Autodesk Inventor part; units mm, degrees
(part 2 of 2)
  spline S96 degree 3 poles (14.7882, -6.4465) (14.7882, -5.3187) (15.0875, -4.3953) (15.6861, -3.6762) knots 0 0 0 0 1 1 1 1
  line L430 (14.7882, -6.4465) -> (14.7882, -5.3187) construction
  line L431 (14.7882, -5.3187) -> (15.0875, -4.3953) construction
  line L432 (15.0875, -4.3953) -> (15.6861, -3.6762) construction
  spline S97 degree 3 poles (15.6861, -3.6762) (16.2847, -2.9572) (17.1023, -2.5977) (18.1388, -2.5977) knots 0 0 0 0 1 1 1 1
  line L433 (15.6861, -3.6762) -> (16.2847, -2.9572) construction
  line L434 (16.2847, -2.9572) -> (17.1023, -2.5977) construction
  line L435 (17.1023, -2.5977) -> (18.1388, -2.5977) construction
  spline S98 degree 3 poles (18.1388, -2.5977) (19.9346, -2.5977) (20.9456, -3.5631) (21.1719, -5.4939) knots 0 0 0 0 1 1 1 1
  line L436 (18.1388, -2.5977) -> (19.9346, -2.5977) construction
  line L437 (19.9346, -2.5977) -> (20.9456, -3.5631) construction
  line L438 (20.9456, -3.5631) -> (21.1719, -5.4939) construction
  line L439 (19.4747, -7.4594) -> (21.1719, -7.5634)
  line L440 (27.9553, -2.7127) -> (27.9553, -10.1858)
  line L441 (27.9553, -10.1858) -> (26.2362, -10.1858)
  line L442 (26.2362, -10.1858) -> (26.2362, -7.1035)
  line L443 (26.2362, -7.1035) -> (23.8984, -7.1035)
  line L444 (23.8984, -7.1035) -> (23.8984, -10.1858)
  line L445 (23.8984, -10.1858) -> (22.1793, -10.1858)
  line L446 (22.1793, -10.1858) -> (22.1793, -2.7127)
  line L447 (22.1793, -2.7127) -> (23.8984, -2.7127)
  line L448 (23.8984, -2.7127) -> (23.8984, -5.6253)
  line L449 (23.8984, -5.6253) -> (26.2362, -5.6253)
  line L450 (26.2362, -5.6253) -> (26.2362, -2.7127)
  line L451 (26.2362, -2.7127) -> (27.9553, -2.7127)
  line L452 (-87.9456, 18.7555) -> (-34.3787, 18.7555) construction
  line L453 (-34.3787, 18.7555) -> (-34.3787, -19.0126) construction
  line L454 (-34.3787, -19.0126) -> (-87.9456, -19.0126) construction
  line L455 (-87.9456, -19.0126) -> (-87.9456, 18.7555) construction
  line L456 (-69.5997, 11.0371) -> (-69.5997, 16.9868)
  line L457 (-69.5997, 16.9868) -> (-68.3878, 16.9868)
  line L458 (-68.3878, 16.9868) -> (-68.3878, 12.0523)
  line L459 (-68.3878, 12.0523) -> (-65.3741, 12.0523)
  line L460 (-65.3741, 12.0523) -> (-65.3741, 11.0371)
  line L461 (-65.3741, 11.0371) -> (-69.5997, 11.0371)
  spline S99 degree 2 poles (-64.7567, 14.0005) (-64.7567, 14.9151) (-64.4823, 15.5371) knots 0 0 0 1 1 1
  spline S100 degree 2 poles (-64.4823, 15.5371) (-64.2765, 15.9944) (-63.5677, 16.7261) (-63.1469, 16.8999) knots 0 0 0 1 2 2 2
  spline S101 degree 2 poles (-63.1469, 16.8999) (-62.589, 17.1377) (-61.8527, 17.1377) knots 0 0 0 1 1 1
  spline S102 degree 2 poles (-61.8527, 17.1377) (-60.5265, 17.1377) (-58.935, 15.4914) (-58.935, 14.0279) knots 0 0 0 1 2 2 2
  spline S103 degree 2 poles (-58.935, 14.0279) (-58.935, 12.5783) (-60.5174, 10.9365) (-61.839, 10.9365) knots 0 0 0 1 2 2 2
  spline S104 degree 2 poles (-61.839, 10.9365) (-63.1744, 10.9365) (-64.7567, 12.5691) (-64.7567, 14.0005) knots 0 0 0 1 2 2 2
  spline S105 degree 2 poles (-63.5082, 14.0417) (-63.5082, 13.0218) (-62.5661, 11.97) (-61.839, 11.97) knots 0 0 0 1 2 2 2
  spline S106 degree 2 poles (-61.839, 11.97) (-61.1119, 11.97) (-60.1835, 13.0127) (-60.1835, 14.0554) knots 0 0 0 1 2 2 2
  spline S107 degree 2 poles (-60.1835, 14.0554) (-60.1835, 15.0889) (-61.089, 16.1042) (-61.839, 16.1042) knots 0 0 0 1 2 2 2
  spline S108 degree 2 poles (-61.839, 16.1042) (-62.589, 16.1042) (-63.5082, 15.0752) (-63.5082, 14.0417) knots 0 0 0 1 2 2 2
  line L462 (-55.1988, 13.2368) -> (-55.1988, 14.252)
  line L463 (-55.1988, 14.252) -> (-52.5875, 14.252)
  line L464 (-52.5875, 14.252) -> (-52.5875, 11.8648)
  spline S109 degree 2 poles (-52.5875, 11.8648) (-52.967, 11.4944) (-54.4122, 10.9365) (-55.153, 10.9365) knots 0 0 0 1 2 2 2
  spline S110 degree 2 poles (-55.153, 10.9365) (-56.0951, 10.9365) (-57.4945, 11.7276) (-58.1988, 13.1956) (-58.1988, 14.0554) knots 0 0 0 1 2 3 3 3
  spline S111 degree 2 poles (-58.1988, 14.0554) (-58.1988, 14.9929) (-57.4122, 16.4517) (-56.6576, 16.8404) knots 0 0 0 1 2 2 2
  spline S112 degree 2 poles (-56.6576, 16.8404) (-56.0768, 17.1377) (-55.217, 17.1377) knots 0 0 0 1 1 1
  spline S113 degree 2 poles (-55.217, 17.1377) (-54.1012, 17.1377) (-52.8436, 16.2002) (-52.6652, 15.3725) knots 0 0 0 1 2 2 2
  line L465 (-52.6652, 15.3725) -> (-53.868, 15.1484)
  spline S114 degree 2 poles (-53.868, 15.1484) (-53.996, 15.592) (-54.6957, 16.1042) (-55.217, 16.1042) knots 0 0 0 1 2 2 2
  spline S115 degree 2 poles (-55.217, 16.1042) (-56.0128, 16.1042) (-56.9503, 15.0981) (-56.9503, 14.1057) knots 0 0 0 1 2 2 2
  spline S116 degree 2 poles (-56.9503, 14.1057) (-56.9503, 13.0401) (-55.9991, 11.97) (-55.2308, 11.97) knots 0 0 0 1 2 2 2
  spline S117 degree 2 poles (-55.2308, 11.97) (-54.8512, 11.97) (-54.0875, 12.2673) (-53.8131, 12.4776) knots 0 0 0 1 2 2 2
  line L466 (-53.8131, 12.4776) -> (-53.8131, 13.2368)
  line L467 (-53.8131, 13.2368) -> (-55.1988, 13.2368)
  line L468 (-80.8131, 1.5949) -> (-80.8131, 7.5949)
  line L469 (-80.8131, 7.5949) -> (-78.8695, 7.5949)
  spline S118 degree 2 poles (-78.8695, 7.5949) (-77.7628, 7.5949) (-77.4289, 7.5034) knots 0 0 0 1 1 1
  spline S119 degree 2 poles (-77.4289, 7.5034) (-76.9122, 7.3708) (-76.217, 6.4653) (-76.217, 5.7473) knots 0 0 0 1 2 2 2
  spline S120 degree 2 poles (-76.217, 5.7473) (-76.217, 5.1985) (-76.6195, 4.444) (-77.2369, 4.0141) (-77.557, 3.9455) knots 0 0 0 1 2 3 3 3
  spline S121 degree 2 poles (-77.557, 3.9455) (-77.9869, 3.8586) (-78.81, 3.8586) knots 0 0 0 1 1 1
  line L470 (-78.81, 3.8586) -> (-79.6012, 3.8586)
  line L471 (-79.6012, 3.8586) -> (-79.6012, 1.5949)
  line L472 (-79.6012, 1.5949) -> (-80.8131, 1.5949)
  line L473 (-79.6012, 6.5796) -> (-79.6012, 4.8738)
  line L474 (-79.6012, 4.8738) -> (-78.9381, 4.8738)
  spline S122 degree 2 poles (-78.9381, 4.8738) (-78.2201, 4.8738) (-77.7399, 5.0613) (-77.4655, 5.4638) (-77.4655, 5.729) knots 0 0 0 1 2 3 3 3
  spline S123 degree 2 poles (-77.4655, 5.729) (-77.4655, 6.0583) (-77.8497, 6.4836) (-78.1469, 6.5385) knots 0 0 0 1 2 2 2
  spline S124 degree 2 poles (-78.1469, 6.5385) (-78.3619, 6.5796) (-79.0158, 6.5796) knots 0 0 0 1 1 1
  line L475 (-79.0158, 6.5796) -> (-79.6012, 6.5796)
  line L476 (-75.2201, 1.5949) -> (-75.2201, 7.5949)
  line L477 (-75.2201, 7.5949) -> (-70.7704, 7.5949)
  line L478 (-70.7704, 7.5949) -> (-70.7704, 6.5796)
  line L479 (-70.7704, 6.5796) -> (-74.0082, 6.5796)
  line L480 (-74.0082, 6.5796) -> (-74.0082, 5.2488)
  line L481 (-74.0082, 5.2488) -> (-70.9945, 5.2488)
  line L482 (-70.9945, 5.2488) -> (-70.9945, 4.2336)
  line L483 (-70.9945, 4.2336) -> (-74.0082, 4.2336)
  line L484 (-74.0082, 4.2336) -> (-74.0082, 2.6101)
  line L485 (-74.0082, 2.6101) -> (-70.6561, 2.6101)
  line L486 (-70.6561, 2.6101) -> (-70.6561, 1.5949)
  line L487 (-70.6561, 1.5949) -> (-75.2201, 1.5949)
  line L488 (-69.6271, 1.5949) -> (-69.6271, 7.5949)
  line L489 (-69.6271, 7.5949) -> (-67.0753, 7.5949)
  spline S125 degree 2 poles (-67.0753, 7.5949) (-66.1103, 7.5949) (-65.2414, 7.2702) (-64.7155, 6.447) (-64.7155, 5.912) knots 0 0 0 1 2 3 3 3
  spline S126 degree 2 poles (-64.7155, 5.912) (-64.7155, 5.2397) (-65.5067, 4.3571) (-66.2978, 4.2427) knots 0 0 0 1 2 2 2
  spline S127 degree 2 poles (-66.2978, 4.2427) (-65.9045, 4.0141) (-65.3924, 3.4653) (-64.9579, 2.7656) knots 0 0 0 1 2 2 2
  line L490 (-64.9579, 2.7656) -> (-64.2262, 1.5949)
  line L491 (-64.2262, 1.5949) -> (-65.6759, 1.5949)
  line L492 (-65.6759, 1.5949) -> (-66.5494, 2.9028)
  spline S128 degree 2 poles (-66.5494, 2.9028) (-67.0204, 3.6025) (-67.3634, 3.9684) (-67.7475, 4.101) (-68.1683, 4.101) knots 0 0 0 1 2 3 3 3
  line L493 (-68.1683, 4.101) -> (-68.4152, 4.101)
  line L494 (-68.4152, 4.101) -> (-68.4152, 1.5949)
  line L495 (-68.4152, 1.5949) -> (-69.6271, 1.5949)
  line L496 (-68.4152, 5.0568) -> (-67.5189, 5.0568)
  spline S129 degree 2 poles (-67.5189, 5.0568) (-66.6454, 5.0568) (-66.2109, 5.2031) (-65.964, 5.5644) (-65.964, 5.8342) knots 0 0 0 1 2 3 3 3
  spline S130 degree 2 poles (-65.964, 5.8342) (-65.964, 6.136) (-66.2887, 6.511) (-66.5814, 6.5613) knots 0 0 0 1 2 2 2
  spline S131 degree 2 poles (-66.5814, 6.5613) (-66.7323, 6.5796) (-67.4686, 6.5796) knots 0 0 0 1 1 1
  line L497 (-67.4686, 6.5796) -> (-68.4152, 6.5796)
  line L498 (-68.4152, 6.5796) -> (-68.4152, 5.0568)
  line L499 (-63.6134, 1.5949) -> (-63.6134, 7.5949)
  line L500 (-63.6134, 7.5949) -> (-62.4015, 7.5949)
  line L501 (-62.4015, 7.5949) -> (-62.4015, 1.5949)
  line L502 (-62.4015, 1.5949) -> (-63.6134, 1.5949)
  spline S132 degree 2 poles (-61.4914, 4.5583) (-61.4914, 5.4729) (-61.217, 6.0949) knots 0 0 0 1 1 1
  spline S133 degree 2 poles (-61.217, 6.0949) (-61.0113, 6.5522) (-60.3024, 7.2839) (-59.8817, 7.4577) knots 0 0 0 1 2 2 2
  spline S134 degree 2 poles (-59.8817, 7.4577) (-59.3238, 7.6955) (-58.5875, 7.6955) knots 0 0 0 1 1 1
  spline S135 degree 2 poles (-58.5875, 7.6955) (-57.2613, 7.6955) (-55.6698, 6.0491) (-55.6698, 4.5857) knots 0 0 0 1 2 2 2
  spline S136 degree 2 poles (-55.6698, 4.5857) (-55.6698, 3.136) (-57.2521, 1.4943) (-58.5738, 1.4943) knots 0 0 0 1 2 2 2
  spline S137 degree 2 poles (-58.5738, 1.4943) (-59.9091, 1.4943) (-61.4914, 3.1269) (-61.4914, 4.5583) knots 0 0 0 1 2 2 2
  spline S138 degree 2 poles (-60.243, 4.5995) (-60.243, 3.5796) (-59.3009, 2.5278) (-58.5738, 2.5278) knots 0 0 0 1 2 2 2
  spline S139 degree 2 poles (-58.5738, 2.5278) (-57.8466, 2.5278) (-56.9183, 3.5705) (-56.9183, 4.6132) knots 0 0 0 1 2 2 2
  spline S140 degree 2 poles (-56.9183, 4.6132) (-56.9183, 5.6467) (-57.8238, 6.662) (-58.5738, 6.662) knots 0 0 0 1 2 2 2
  spline S141 degree 2 poles (-58.5738, 6.662) (-59.3238, 6.662) (-60.243, 5.633) (-60.243, 4.5995) knots 0 0 0 1 2 2 2
  line L503 (-54.7323, 7.5949) -> (-52.5143, 7.5949)
  spline S142 degree 2 poles (-52.5143, 7.5949) (-51.7643, 7.5949) (-51.371, 7.4805) knots 0 0 0 1 1 1
  spline S143 degree 2 poles (-51.371, 7.4805) (-50.8451, 7.3251) (-50.0905, 6.5293) (-49.6972, 5.3815) (-49.6972, 4.5354) knots 0 0 0 1 2 3 3 3
  spline S144 degree 2 poles (-49.6972, 4.5354) (-49.6972, 3.7946) (-49.8802, 3.2595) knots 0 0 0 1 1 1
  spline S145 degree 2 poles (-49.8802, 3.2595) (-50.1088, 2.6055) (-50.525, 2.1985) knots 0 0 0 1 1 1
  spline S146 degree 2 poles (-50.525, 2.1985) (-50.8405, 1.8921) (-51.3756, 1.7229) knots 0 0 0 1 1 1
  spline S147 degree 2 poles (-51.3756, 1.7229) (-51.778, 1.5949) (-52.4503, 1.5949) knots 0 0 0 1 1 1
  line L504 (-52.4503, 1.5949) -> (-54.7323, 1.5949)
  line L505 (-54.7323, 1.5949) -> (-54.7323, 7.5949)
  line L506 (-53.5204, 6.5796) -> (-53.5204, 2.6101)
  line L507 (-53.5204, 2.6101) -> (-52.6149, 2.6101)
  spline S148 degree 2 poles (-52.6149, 2.6101) (-52.1027, 2.6101) (-51.8786, 2.6696) knots 0 0 0 1 1 1
  spline S149 degree 2 poles (-51.8786, 2.6696) (-51.5814, 2.7427) (-51.1927, 3.0903) (-50.9457, 3.8998) (-50.9457, 4.5949) knots 0 0 0 1 2 3 3 3
  spline S150 degree 2 poles (-50.9457, 4.5949) (-50.9457, 5.29) (-51.1927, 6.0309) (-51.6363, 6.447) (-51.9747, 6.5202) knots 0 0 0 1 2 3 3 3
  spline S151 degree 2 poles (-51.9747, 6.5202) (-52.2308, 6.5796) (-52.9762, 6.5796) knots 0 0 0 1 1 1
  line L508 (-52.9762, 6.5796) -> (-53.5204, 6.5796)
  line L509 (-48.7094, 1.5949) -> (-48.7094, 7.5949)
  line L510 (-48.7094, 7.5949) -> (-47.4975, 7.5949)
  line L511 (-47.4975, 7.5949) -> (-47.4975, 1.5949)
  line L512 (-47.4975, 1.5949) -> (-48.7094, 1.5949)
  line L513 (-42.5036, 3.8037) -> (-41.3283, 3.4333)
  spline S152 degree 2 poles (-41.3283, 3.4333) (-41.5981, 2.4501) (-42.8558, 1.4943) (-43.8207, 1.4943) knots 0 0 0 1 2 2 2
  spline S153 degree 2 poles (-43.8207, 1.4943) (-45.0143, 1.4943) (-46.5555, 3.1269) (-46.5555, 4.54) knots 0 0 0 1 2 2 2
  spline S154 degree 2 poles (-46.5555, 4.54) (-46.5555, 6.04) (-45.0097, 7.6955) (-43.7475, 7.6955) knots 0 0 0 1 2 2 2
  spline S155 degree 2 poles (-43.7475, 7.6955) (-42.65, 7.6955) (-41.9594, 7.0461) knots 0 0 0 1 1 1
  spline S156 degree 2 poles (-41.9594, 7.0461) (-41.5524, 6.662) (-41.3466, 5.944) knots 0 0 0 1 1 1
  line L514 (-41.3466, 5.944) -> (-42.5448, 5.6559)
  spline S157 degree 2 poles (-42.5448, 5.6559) (-42.65, 6.1223) (-43.3268, 6.662) (-43.807, 6.662) knots 0 0 0 1 2 2 2
  spline S158 degree 2 poles (-43.807, 6.662) (-44.4747, 6.662) (-45.307, 5.7062) (-45.307, 4.6315) knots 0 0 0 1 2 2 2
  spline S159 degree 2 poles (-45.307, 4.6315) (-45.307, 3.4927) (-44.4884, 2.5278) (-43.8344, 2.5278) knots 0 0 0 1 2 2 2
  spline S160 degree 2 poles (-43.8344, 2.5278) (-43.3497, 2.5278) (-42.6545, 3.1452) (-42.5036, 3.8037) knots 0 0 0 1 2 2 2
  line L515 (-75.6385, -7.8473) -> (-76.9556, -7.8473)
  line L516 (-76.9556, -7.8473) -> (-77.477, -6.4845)
  line L517 (-77.477, -6.4845) -> (-79.8733, -6.4845)
  line L518 (-79.8733, -6.4845) -> (-80.3718, -7.8473)
  line L519 (-80.3718, -7.8473) -> (-81.6568, -7.8473)
  line L520 (-81.6568, -7.8473) -> (-79.3245, -1.8473)
  line L521 (-79.3245, -1.8473) -> (-78.0349, -1.8473)
  line L522 (-78.0349, -1.8473) -> (-75.6385, -7.8473)
  line L523 (-77.8657, -5.4693) -> (-78.6934, -3.2467)
  line L524 (-78.6934, -3.2467) -> (-79.5074, -5.4693)
  line L525 (-79.5074, -5.4693) -> (-77.8657, -5.4693)
  line L526 (-74.98, -7.8473) -> (-74.98, -1.8473)
  line L527 (-74.98, -1.8473) -> (-73.8047, -1.8473)
  line L528 (-73.8047, -1.8473) -> (-71.3398, -5.8717)
  line L529 (-71.3398, -5.8717) -> (-71.3398, -1.8473)
  line L530 (-71.3398, -1.8473) -> (-70.2193, -1.8473)
  line L531 (-70.2193, -1.8473) -> (-70.2193, -7.8473)
  line L532 (-70.2193, -7.8473) -> (-71.4312, -7.8473)
  line L533 (-71.4312, -7.8473) -> (-73.8596, -3.9098)
  line L534 (-73.8596, -3.9098) -> (-73.8596, -7.8473)
  line L535 (-73.8596, -7.8473) -> (-74.98, -7.8473)
  line L536 (-67.5852, -7.8473) -> (-67.5852, -2.8626)
  line L537 (-67.5852, -2.8626) -> (-69.3641, -2.8626)
  line L538 (-69.3641, -2.8626) -> (-69.3641, -1.8473)
  line L539 (-69.3641, -1.8473) -> (-64.5989, -1.8473)
  line L540 (-64.5989, -1.8473) -> (-64.5989, -2.8626)
  line L541 (-64.5989, -2.8626) -> (-66.3733, -2.8626)
  line L542 (-66.3733, -2.8626) -> (-66.3733, -7.8473)
  line L543 (-66.3733, -7.8473) -> (-67.5852, -7.8473)
  line L544 (-63.8123, -7.8473) -> (-63.8123, -1.8473)
  line L545 (-63.8123, -1.8473) -> (-59.3626, -1.8473)
  line L546 (-59.3626, -1.8473) -> (-59.3626, -2.8626)
  line L547 (-59.3626, -2.8626) -> (-62.6004, -2.8626)
  line L548 (-62.6004, -2.8626) -> (-62.6004, -4.1934)
  line L549 (-62.6004, -4.1934) -> (-59.5867, -4.1934)
  line L550 (-59.5867, -4.1934) -> (-59.5867, -5.2086)
  line L551 (-59.5867, -5.2086) -> (-62.6004, -5.2086)
  line L552 (-62.6004, -5.2086) -> (-62.6004, -6.8321)
  line L553 (-62.6004, -6.8321) -> (-59.2483, -6.8321)
  line L554 (-59.2483, -6.8321) -> (-59.2483, -7.8473)
  line L555 (-59.2483, -7.8473) -> (-63.8123, -7.8473)
  line L556 (-58.2102, -7.8473) -> (-58.2102, -1.8473)
  line L557 (-58.2102, -1.8473) -> (-57.0349, -1.8473)
  line L558 (-57.0349, -1.8473) -> (-54.5699, -5.8717)
  line L559 (-54.5699, -5.8717) -> (-54.5699, -1.8473)
  line L560 (-54.5699, -1.8473) -> (-53.4495, -1.8473)
  line L561 (-53.4495, -1.8473) -> (-53.4495, -7.8473)
  line L562 (-53.4495, -7.8473) -> (-54.6614, -7.8473)
  line L563 (-54.6614, -7.8473) -> (-57.0898, -3.9098)
  line L564 (-57.0898, -3.9098) -> (-57.0898, -7.8473)
  line L565 (-57.0898, -7.8473) -> (-58.2102, -7.8473)
  line L566 (-52.1553, -7.8473) -> (-52.1553, -1.8473)
  line L567 (-52.1553, -1.8473) -> (-50.98, -1.8473)
  line L568 (-50.98, -1.8473) -> (-48.5151, -5.8717)
  line L569 (-48.5151, -5.8717) -> (-48.5151, -1.8473)
  line L570 (-48.5151, -1.8473) -> (-47.3946, -1.8473)
  line L571 (-47.3946, -1.8473) -> (-47.3946, -7.8473)
  line L572 (-47.3946, -7.8473) -> (-48.6065, -7.8473)
  line L573 (-48.6065, -7.8473) -> (-51.0349, -3.9098)
  line L574 (-51.0349, -3.9098) -> (-51.0349, -7.8473)
  line L575 (-51.0349, -7.8473) -> (-52.1553, -7.8473)
  line L576 (-40.7041, -7.8473) -> (-42.0212, -7.8473)
  line L577 (-42.0212, -7.8473) -> (-42.5425, -6.4845)
  line L578 (-42.5425, -6.4845) -> (-44.9388, -6.4845)
  line L579 (-44.9388, -6.4845) -> (-45.4373, -7.8473)
  line L580 (-45.4373, -7.8473) -> (-46.7224, -7.8473)
  line L581 (-46.7224, -7.8473) -> (-44.3901, -1.8473)
  line L582 (-44.3901, -1.8473) -> (-43.1004, -1.8473)
  line L583 (-43.1004, -1.8473) -> (-40.7041, -7.8473)
  line L584 (-42.9312, -5.4693) -> (-43.759, -3.2467)
  line L585 (-43.759, -3.2467) -> (-44.573, -5.4693)
  line L586 (-44.573, -5.4693) -> (-42.9312, -5.4693)
  spline S161 degree 2 poles (-80.2872, -11.2667) (-79.4137, -11.2667) (-78.9244, -11.8886) knots 0 0 0 1 1 1
  spline S162 degree 2 poles (-78.9244, -11.8886) (-78.339, -12.6249) (-78.339, -14.3307) knots 0 0 0 1 1 1
  spline S163 degree 2 poles (-78.339, -14.3307) (-78.339, -16.0319) (-78.9289, -16.7774) knots 0 0 0 1 1 1
  spline S164 degree 2 poles (-78.9289, -16.7774) (-79.4137, -17.3902) (-80.2872, -17.3902) knots 0 0 0 1 1 1
  spline S165 degree 2 poles (-80.2872, -17.3902) (-81.1652, -17.3902) (-82.2353, -16.0456) (-82.2353, -14.317) knots 0 0 0 1 2 2 2
  spline S166 degree 2 poles (-82.2353, -14.317) (-82.2353, -12.6249) (-81.6454, -11.8795) knots 0 0 0 1 1 1
  spline S167 degree 2 poles (-81.6454, -11.8795) (-81.1606, -11.2667) (-80.2872, -11.2667) knots 0 0 0 1 1 1
  spline S168 degree 2 poles (-80.2872, -12.2225) (-80.4975, -12.2225) (-80.8222, -12.4877) (-80.9137, -12.8307) knots 0 0 0 1 2 2 2
  spline S169 degree 2 poles (-80.9137, -12.8307) (-81.0326, -13.2743) (-81.0326, -14.3307) knots 0 0 0 1 1 1
  spline S170 degree 2 poles (-81.0326, -14.3307) (-81.0326, -15.3825) (-80.8177, -16.1737) (-80.4975, -16.4344) (-80.2872, -16.4344) knots 0 0 0 1 2 3 3 3
  spline S171 degree 2 poles (-80.2872, -16.4344) (-80.0768, -16.4344) (-79.7521, -16.1691) (-79.6606, -15.8261) knots 0 0 0 1 2 2 2
  spline S172 degree 2 poles (-79.6606, -15.8261) (-79.5417, -15.3825) (-79.5417, -14.3307) knots 0 0 0 1 1 1
  spline S173 degree 2 poles (-79.5417, -14.3307) (-79.5417, -13.2743) (-79.7567, -12.4877) (-80.0768, -12.2225) (-80.2872, -12.2225) knots 0 0 0 1 2 3 3 3
  line L587 (-77.3283, -17.2896) -> (-77.3283, -16.1371)
  line L588 (-77.3283, -16.1371) -> (-76.1759, -16.1371)
  line L589 (-76.1759, -16.1371) -> (-76.1759, -17.2896)
  line L590 (-76.1759, -17.2896) -> (-77.3283, -17.2896)
  spline S174 degree 2 poles (-74.2597, -14.0517) (-74.7033, -13.8642) (-75.1103, -13.2057) (-75.1103, -12.8124) knots 0 0 0 1 2 2 2
  spline S175 degree 2 poles (-75.1103, -12.8124) (-75.1103, -12.1402) (-74.1728, -11.2667) (-73.3085, -11.2667) knots 0 0 0 1 2 2 2
  spline S176 degree 2 poles (-73.3085, -11.2667) (-72.4533, -11.2667) (-71.5067, -12.1402) (-71.5067, -12.8124) knots 0 0 0 1 2 2 2
  spline S177 degree 2 poles (-71.5067, -12.8124) (-71.5067, -13.2286) (-71.9411, -13.878) (-72.3344, -14.0517) knots 0 0 0 1 2 2 2
  spline S178 degree 2 poles (-72.3344, -14.0517) (-71.8359, -14.253) (-71.3146, -15.0213) (-71.3146, -15.5243) knots 0 0 0 1 2 2 2
  spline S179 degree 2 poles (-71.3146, -15.5243) (-71.3146, -16.3566) (-72.3756, -17.3947) (-73.2536, -17.3947) knots 0 0 0 1 2 2 2
  spline S180 degree 2 poles (-73.2536, -17.3947) (-74.0722, -17.3947) (-74.6164, -16.9649) knots 0 0 0 1 1 1
  spline S181 degree 2 poles (-74.6164, -16.9649) (-75.2613, -16.4572) (-75.2613, -15.5746) knots 0 0 0 1 1 1
  spline S182 degree 2 poles (-75.2613, -15.5746) (-75.2613, -15.0853) (-74.7765, -14.2713) (-74.2597, -14.0517) knots 0 0 0 1 2 2 2
  spline S183 degree 2 poles (-74.1271, -15.4649) (-74.1271, -15.9405) (-73.6424, -16.471) (-73.2765, -16.471) knots 0 0 0 1 2 2 2
  spline S184 degree 2 poles (-73.2765, -16.471) (-72.9198, -16.471) (-72.4533, -15.9588) (-72.4533, -15.474) knots 0 0 0 1 2 2 2
  spline S185 degree 2 poles (-72.4533, -15.474) (-72.4533, -15.0533) (-72.9289, -14.5411) (-73.2902, -14.5411) knots 0 0 0 1 2 2 2
  spline S186 degree 2 poles (-73.2902, -14.5411) (-73.7155, -14.5411) (-74.1271, -15.1219) (-74.1271, -15.4649) knots 0 0 0 1 2 2 2
  spline S187 degree 2 poles (-74.0219, -12.8947) (-74.0219, -13.2377) (-73.6332, -13.6219) (-73.3085, -13.6219) knots 0 0 0 1 2 2 2
  spline S188 degree 2 poles (-73.3085, -13.6219) (-72.9792, -13.6219) (-72.5859, -13.2331) (-72.5859, -12.8902) knots 0 0 0 1 2 2 2
  spline S189 degree 2 poles (-72.5859, -12.8902) (-72.5859, -12.57) (-72.9747, -12.1813) (-73.2948, -12.1813) knots 0 0 0 1 2 2 2
  spline S190 degree 2 poles (-73.2948, -12.1813) (-73.6286, -12.1813) (-74.0219, -12.5746) (-74.0219, -12.8947) knots 0 0 0 1 2 2 2
  line L591 (-68.1408, -15.6889) -> (-68.1408, -14.5365)
  line L592 (-68.1408, -14.5365) -> (-65.8817, -14.5365)
  line L593 (-65.8817, -14.5365) -> (-65.8817, -15.6889)
  line L594 (-65.8817, -15.6889) -> (-68.1408, -15.6889)
  line L595 (-59.2414, -12.7575) -> (-60.3527, -12.881)
  spline S191 degree 2 poles (-60.3527, -12.881) (-60.3939, -12.538) (-60.7369, -12.2133) (-61.0113, -12.2133) knots 0 0 0 1 2 2 2
  spline S192 degree 2 poles (-61.0113, -12.2133) (-61.3771, -12.2133) (-61.8802, -12.8673) (-61.9442, -13.9008) knots 0 0 0 1 2 2 2
  spline S193 degree 2 poles (-61.9442, -13.9008) (-61.5189, -13.3932) (-60.8786, -13.3932) knots 0 0 0 1 1 1
  spline S194 degree 2 poles (-60.8786, -13.3932) (-60.1606, -13.3932) (-59.1317, -14.4908) (-59.1317, -15.3551) knots 0 0 0 1 2 2 2
  spline S195 degree 2 poles (-59.1317, -15.3551) (-59.1317, -16.2789) (-60.2109, -17.3902) (-61.057, -17.3902) knots 0 0 0 1 2 2 2
  spline S196 degree 2 poles (-61.057, -17.3902) (-61.967, -17.3902) (-63.1378, -15.9771) (-63.1378, -14.3719) knots 0 0 0 1 2 2 2
  spline S197 degree 2 poles (-63.1378, -14.3719) (-63.1378, -12.721) (-61.9167, -11.2667) (-60.9427, -11.2667) knots 0 0 0 1 2 2 2
  spline S198 degree 2 poles (-60.9427, -11.2667) (-60.2613, -11.2667) (-59.3649, -12.0304) (-59.2414, -12.7575) knots 0 0 0 1 2 2 2
  spline S199 degree 2 poles (-61.8481, -15.2636) (-61.8481, -15.8261) (-61.3314, -16.4344) (-61.0021, -16.4344) knots 0 0 0 1 2 2 2
  spline S200 degree 2 poles (-61.0021, -16.4344) (-60.682, -16.4344) (-60.2567, -15.9359) (-60.2567, -15.3688) knots 0 0 0 1 2 2 2
  spline S201 degree 2 poles (-60.2567, -15.3688) (-60.2567, -14.7835) (-60.714, -14.2392) (-61.057, -14.2392) knots 0 0 0 1 2 2 2
  spline S202 degree 2 poles (-61.057, -14.2392) (-61.3908, -14.2392) (-61.8481, -14.7606) (-61.8481, -15.2636) knots 0 0 0 1 2 2 2
  line L596 (-53.1042, -15.0899) -> (-53.1042, -14.0746)
  line L597 (-53.1042, -14.0746) -> (-50.493, -14.0746)
  line L598 (-50.493, -14.0746) -> (-50.493, -16.4618)
  spline S203 degree 2 poles (-50.493, -16.4618) (-50.8725, -16.8322) (-52.3177, -17.3902) (-53.0585, -17.3902) knots 0 0 0 1 2 2 2
  spline S204 degree 2 poles (-53.0585, -17.3902) (-54.0006, -17.3902) (-55.4, -16.599) (-56.1042, -15.131) (-56.1042, -14.2713) knots 0 0 0 1 2 3 3 3
  spline S205 degree 2 poles (-56.1042, -14.2713) (-56.1042, -13.3338) (-55.3177, -11.8749) (-54.5631, -11.4862) knots 0 0 0 1 2 2 2
  spline S206 degree 2 poles (-54.5631, -11.4862) (-53.9823, -11.1889) (-53.1225, -11.1889) knots 0 0 0 1 1 1
  spline S207 degree 2 poles (-53.1225, -11.1889) (-52.0067, -11.1889) (-50.7491, -12.1264) (-50.5707, -12.9542) knots 0 0 0 1 2 2 2
  line L599 (-50.5707, -12.9542) -> (-51.7734, -13.1783)
  spline S208 degree 2 poles (-51.7734, -13.1783) (-51.9015, -12.7347) (-52.6012, -12.2225) (-53.1225, -12.2225) knots 0 0 0 1 2 2 2
  spline S209 degree 2 poles (-53.1225, -12.2225) (-53.9183, -12.2225) (-54.8558, -13.2286) (-54.8558, -14.221) knots 0 0 0 1 2 2 2
  spline S210 degree 2 poles (-54.8558, -14.221) (-54.8558, -15.2865) (-53.9045, -16.3566) (-53.1363, -16.3566) knots 0 0 0 1 2 2 2
  spline S211 degree 2 poles (-53.1363, -16.3566) (-52.7567, -16.3566) (-51.993, -16.0594) (-51.7186, -15.849) knots 0 0 0 1 2 2 2
  line L600 (-51.7186, -15.849) -> (-51.7186, -15.0899)
  line L601 (-51.7186, -15.0899) -> (-53.1042, -15.0899)
  line L602 (-49.3725, -17.2896) -> (-49.3725, -11.2896)
  line L603 (-49.3725, -11.2896) -> (-48.1606, -11.2896)
  line L604 (-48.1606, -11.2896) -> (-48.1606, -13.6493)
  line L605 (-48.1606, -13.6493) -> (-45.7872, -13.6493)
  line L606 (-45.7872, -13.6493) -> (-45.7872, -11.2896)
  line L607 (-45.7872, -11.2896) -> (-44.5753, -11.2896)
  line L608 (-44.5753, -11.2896) -> (-44.5753, -17.2896)
  line L609 (-44.5753, -17.2896) -> (-45.7872, -17.2896)
  line L610 (-45.7872, -17.2896) -> (-45.7872, -14.6646)
  line L611 (-45.7872, -14.6646) -> (-48.1606, -14.6646)
  line L612 (-48.1606, -14.6646) -> (-48.1606, -17.2896)
  line L613 (-48.1606, -17.2896) -> (-49.3725, -17.2896)
  line L614 (-43.7933, -17.2896) -> (-43.7933, -16.3841)
  line L615 (-43.7933, -16.3841) -> (-42.1652, -14.5228)
  spline S212 degree 2 poles (-42.1652, -14.5228) (-41.7628, -14.0655) (-41.5707, -13.8734) knots 0 0 0 1 1 1
  spline S213 degree 2 poles (-41.5707, -13.8734) (-41.7719, -13.8825) (-42.0966, -13.8871) knots 0 0 0 1 1 1
  line L616 (-42.0966, -13.8871) -> (-43.6332, -13.8963)
  line L617 (-43.6332, -13.8963) -> (-43.6332, -12.9405)
  line L618 (-43.6332, -12.9405) -> (-40.0387, -12.9405)
  line L619 (-40.0387, -12.9405) -> (-40.0387, -13.7591)
  line L620 (-40.0387, -13.7591) -> (-41.7033, -15.6706)
  line L621 (-41.7033, -15.6706) -> (-42.2887, -16.3017)
  spline S214 degree 2 poles (-42.2887, -16.3017) (-41.8085, -16.2789) (-41.6942, -16.2789) knots 0 0 0 1 1 1
  line L622 (-41.6942, -16.2789) -> (-39.9106, -16.2789)
  line L623 (-39.9106, -16.2789) -> (-39.9106, -17.2896)
  line L624 (-39.9106, -17.2896) -> (-43.7933, -17.2896)
  point P0 (0, 0)
  point P1 (27.7034, 2.3054)
  point P2 (29.7605, 2.9065)
  point P3 (30.0143, 5.4965)
  point P4 (28.8487, 6.1923)
  point P5 (30.1945, 7.8509)
  point P6 (29.888, 8.8915)
  point P7 (27.3201, 3.6906)
  point P8 (27.3914, 5.4918)
  point P9 (28.5739, 4.5986)
  point P10 (27.899, 8.4049)
  point P11 (28.2071, 7.1069)
  point P12 (23.4166, 2.3054)
  point P13 (6.2091, 2.3054)
  point P14 (10.266, 2.3054)
  point P15 (0.4496, 9.8936)
  point P16 (-2.901, 6.0448)
  point P17 (0.4379, 2.1905)
  point P18 (2.4808, 2.8858)
  point P19 (1.7855, 5.0319)
  point P20 (0.4671, 3.6194)
  point P21 (-0.5797, 4.1176)
  point P22 (-0.952, 6.0283)
  point P23 (0.4167, 8.4646)
  point P24 (-11.5349, 2.3054)
  point P25 (-17.7433, 2.3054)
  point P26 (-24.5157, 2.3054)
  point P27 (-22.4587, 2.9065)
  point P28 (-22.2048, 5.4965)
  point P29 (-23.3704, 6.1923)
  point P30 (-22.0247, 7.8509)
  point P31 (-22.3312, 8.8915)
  point P32 (-23.1087, 9.5487)
  point P33 (-24.8278, 5.4918)
  point P34 (-24.3202, 8.4049)
  point P35 (-23.8204, 7.6598)
  point P36 (-24.0121, 7.1069)
  point P37 (22.1793, -2.7127)
  point P38 (18.1564, -8.8719)
  point P39 (19.4747, -7.4594)
  point P40 (18.1271, -10.3008)
  point P41 (15.6861, -3.6762)
  point P42 (18.1388, -2.5977)
  point P43 (12.6729, -2.9296)
  point P44 (13.5783, -3.6981)
  point P45 (13.9396, -4.9519)
  point P46 (7.9228, -2.7127)
  point P47 (2.749, -2.7127)
  point P48 (-0.7056, -5.6691)
  point P49 (0.0554, -8.7076)
  point P50 (-5.2881, -2.7127)
  point P51 (0.0554, -2.7127)
  point P52 (-10.4344, -4.64)
  point P53 (-10.2359, -5.1006)
  point P54 (-9.356, -5.4183)
  point P55 (-7.686, -5.8826)
  point P56 (-6.7896, -6.6493)
  point P57 (-9.5201, -10.3008)
  point P58 (-11.4827, -9.779)
  point P59 (-9.3997, -8.9047)
  point P60 (-9.5177, -7.266)
  point P61 (-11.549, -6.4602)
  point P62 (-12.1535, -4.9622)
  point P63 (-9.4599, -2.5977)
  point P64 (-18.1868, -2.7127)
  point P65 (-20.8003, -2.9296)
  point P66 (-19.895, -3.6981)
  point P67 (-25.5505, -2.7127)
  point P68 (11.5275, -5.8746)
  point P69 (11.9489, -5.5457)
  point P70 (11.9468, -4.4044)
  point P71 (-21.9457, -5.8746)
  point P72 (-21.5244, -5.5457)
  point P73 (-21.5265, -4.4044)
  dimension "d72" = 6.9444
  dimension "d73" = 6.381
  constraints: 310 end point, 299 other
  measures "d72" distance between parallel lines of L219 L453
  measures "d73" distance between parallel lines of L453 L26
extrude "Extrusion6" cut sketch "Sketch6" against normal blind 1
sketch "Sketch7" plane through (-118.515, -0.5568, -11.175) normal (1, 0, 0) x (0, 0, -1)
  arc A0 (0, 3.15) -> (0, -3.15) centre (0, 0) ccw projected
  line L0 (-2.4537, -4.25) -> (-4.9075, 0)
  line L1 (-4.9075, 0) -> (-2.4537, 4.25)
  line L2 (-2.4537, 4.25) -> (2.4537, 4.25)
  line L3 (2.4537, 4.25) -> (4.9075, 0)
  line L4 (4.9075, 0) -> (2.4537, -4.25)
  line L5 (2.4537, -4.25) -> (-2.4537, -4.25)
  point P0 (-11.175, 0.5568)
  dimension "d76" = 8.5
  constraints: 12 end point, 1 coincident, 13 other
  measures "d76" distance between parallel lines of L5 L2
extrude "Extrusion7" cut sketch "Sketch7" against normal blind 1
equation "\"d25\" = d24"
equation "\"d26\" = d24"
equation "\"d27\" = d24"
equation "\"d28\" = d24"
equation "\"d29\" = d24"
equation "\"d40\" = 0.5 * d39"
equation "\"d67\" = d66"
equation "\"d68\" = d66"
equation "\"d69\" = d66"
equation "\"d70\" = d66"
equation "\"d71\" = d66"
body "Solid1"
